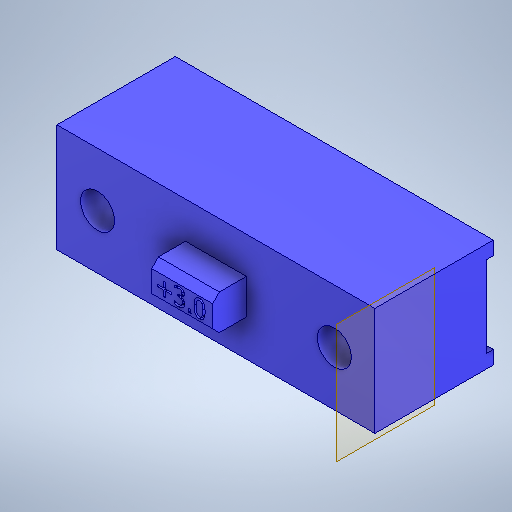
# Autodesk Inventor part: Bearing Spacer_V2_3mm
Saved by Autodesk Inventor 2025.4 (Build 294407000, 407)
## iProperties
Created: 2026-06-01
Part Number: Bearing Spacer_V2_3mm
Material: 일반
Document SubType Name: Modeling
Designer: dalbi
Density: 1 g/cm^3
Appearance: 기본값
Author: dalbi
Autodesk Inventor part; units mm, degrees
ref_plane "YZ Plane" through (0, 0, 0) normal (1, 0, 0) x (0, 1, 0)
ref_plane "XZ Plane" through (0, 0, 0) normal (0, 1, 0) x (-1, 0, 0)
ref_plane "XY Plane" through (0, 0, 0) normal (0, 0, 1) x (1, 0, 0)
ref_plane "작업 평면1" through (23.5, -8, -2) normal (1, 0, 0) x (0, 0, -1)
sketch "스케치1" plane through (23.5, -8, -2) normal (1, 0, 0) x (0, 0, -1)
  line L0 (0, 16) -> (-8.15, 16) projected
  line L1 (-8.15, 16) -> (-8.15, 10.6) projected
  line L2 (-8.15, 10.6) -> (-12.15, 10.6) projected
  line L3 (-13.15, 9.6) -> (-12.15, 10.6) projected
  line L4 (-13.15, 9.6) -> (-13.15, 6.4) projected
  line L5 (-12.15, 5.4) -> (-13.15, 6.4) projected
  line L6 (-12.15, 5.4) -> (-8.15, 5.4) projected
  line L7 (-8.15, 5.4) -> (-8.15, 0) projected
  line L8 (-8.15, 0) -> (0, 0) projected
  line L9 (0, 16) -> (9.35, 16)
  line L10 (9.35, 16) -> (9.35, 15)
  line L11 (0, 0) -> (9.35, 0)
  line L12 (9.35, 0) -> (9.35, 1)
  line L13 (0, 16) -> (-8.15, 16)
  line L14 (-8.15, 10.6) -> (-12.15, 10.6) projected
  line L15 (-8.15, 10.6) -> (-12.15, 10.6)
  line L16 (-12.15, 10.6) -> (-13.15, 9.6)
  line L17 (-13.15, 6.4) -> (-12.15, 5.4)
  line L18 (8.35, 14) -> (9.35, 14)
  line L19 (9.35, 14) -> (9.35, 15)
  line L20 (8.35, 2) -> (9.35, 2)
  line L21 (9.35, 2) -> (9.35, 1)
  line L22 (8.35, 14) -> (8.35, 2)
  point P0 (-2, 8)
  point P1 (4.35, 10.6)
  point P2 (4.35, 5.4)
  dimension "d1" = 9.35
  dimension "d13" = 9.35
  constraints: 26 end point, 5 perpendicular, 4 horizontal, 2 collinear, 2 point on line
  measures "d1" distance of L0.start L9.end
  measures "d13" distance of L8.end L11.end
sketch "스케치2" plane through (-23.5, 8, 6.15) normal (0, 0, 1) x (1, 0, 0)
  arc A0 (7.9209, -9.6) -> (7.9209, -6.4) centre (6, -8) ccw projected
  line L0 (39.0791, -9.6) -> (7.9209, -9.6) projected
  circle A1 centre (6, -8) radius 2.5
  circle A2 centre (41, -8) radius 2.5 projected
  circle A3 centre (41, -8) radius 2.5
  point P0 (23.5, -8)
  point P1 (7.9209, -6.4)
  constraints: 2 coincident, 1 centre point, 4 other
extrude "돌출1" add sketch "스케치1" against normal up to surface (47 mm away)
extrude "돌출2" cut sketch "스케치2" along normal mid plane 50
sketch "스케치3" plane through (-15.5791, 1.6, 11.15) normal (0, 0, 1) x (1, 0, 0)
  line L0 (15.5791, -14.4593) -> (15.5791, 15.5737)
  line L1 (-7.9209, 4.4) -> (-7.9209, -7.6) projected
  line L2 (-7.9209, 4.4) -> (11.0791, 4.4)
  line L3 (11.0791, 4.4) -> (11.0791, -7.6)
  line L4 (11.0791, -7.6) -> (-7.9209, -7.6)
  line L5 (-7.9209, -7.6) -> (-7.9209, 4.4)
  line L6 (39.0791, 4.4) -> (39.0791, -7.6)
  line L7 (39.0791, 4.4) -> (20.0791, 4.4)
  line L8 (20.0791, 4.4) -> (20.0791, -7.6)
  line L9 (20.0791, -7.6) -> (39.0791, -7.6)
  line L10 (39.0791, -7.6) -> (39.0791, 4.4)
  point P0 (15.5791, -1.6)
  dimension "d9" = 19
  constraints: 20 end point, 5 symmetric about line, 2 parallel, 1 horizontal, 1 perpendicular, 1 vertical
  measures "d9" distance of L1.start L2.end
extrude "돌출3" cut sketch "스케치3" against normal up to surface (5 mm away)
sketch "스케치4" plane through (-4.5, 1.6, 11.15) normal (0, 0, 1) x (1, 0, 0)
  line L0 (0.6181, -0.2528) -> (7.2489, -0.2528) construction
  line L1 (7.2489, -0.2528) -> (7.2489, -2.6222) construction
  line L2 (7.2489, -2.6222) -> (0.6181, -2.6222) construction
  line L3 (0.6181, -2.6222) -> (0.6181, -0.2528) construction
  line L4 (2.8925, -1.8707) -> (2.0321, -1.8707)
  line L5 (2.0321, -1.8707) -> (2.0321, -2.7311)
  line L6 (2.0321, -2.7311) -> (1.7481, -2.7311)
  line L7 (1.7481, -2.7311) -> (1.7481, -1.8707)
  line L8 (1.7481, -1.8707) -> (0.8877, -1.8707)
  line L9 (0.8877, -1.8707) -> (0.8877, -1.5969)
  line L10 (0.8877, -1.5969) -> (1.7481, -1.5969)
  line L11 (1.7481, -1.5969) -> (1.7481, -0.7365)
  line L12 (1.7481, -0.7365) -> (2.0321, -0.7365)
  line L13 (2.0321, -0.7365) -> (2.0321, -1.5969)
  line L14 (2.0321, -1.5969) -> (2.8925, -1.5969)
  line L15 (2.8925, -1.5969) -> (2.8925, -1.8707)
  spline S0 degree 2 poles (4.0308, -0.5472) (3.9382, -0.5472) (3.755, -0.5925) (3.6665, -0.6274) knots 0 0 0 1 2 2 2
  spline S1 degree 2 poles (3.6665, -0.6274) (3.5841, -0.6624) (3.4627, -0.7365) (3.4154, -0.7695) knots 0 0 0 1 2 2 2
  line L16 (3.4154, -0.7695) -> (3.3948, -0.7695)
  line L17 (3.3948, -0.7695) -> (3.3948, -0.4093)
  spline S2 degree 2 poles (3.3948, -0.4093) (3.5059, -0.3496) (3.8867, -0.2528) (4.0576, -0.2528) knots 0 0 0 1 2 2 2
  spline S3 degree 2 poles (4.0576, -0.2528) (4.2305, -0.2528) (4.4878, -0.3228) (4.5927, -0.3969) knots 0 0 0 1 2 2 2
  spline S4 degree 2 poles (4.5927, -0.3969) (4.7039, -0.4772) (4.8191, -0.7098) (4.8191, -0.8662) knots 0 0 0 1 2 2 2
  spline S5 degree 2 poles (4.8191, -0.8662) (4.8191, -1.0762) (4.5433, -1.3932) (4.3498, -1.4343) knots 0 0 0 1 2 2 2
  line L18 (4.3498, -1.4343) -> (4.3498, -1.459)
  spline S6 degree 2 poles (4.3498, -1.459) (4.4301, -1.4755) (4.6133, -1.5496) (4.6915, -1.6237) knots 0 0 0 1 2 2 2
  spline S7 degree 2 poles (4.6915, -1.6237) (4.7697, -1.6957) (4.8685, -1.9263) (4.8685, -2.093) knots 0 0 0 1 2 2 2
  spline S8 degree 2 poles (4.8685, -2.093) (4.8685, -2.2638) (4.7512, -2.5541) (4.6442, -2.6652) knots 0 0 0 1 2 2 2
  spline S9 degree 2 poles (4.6442, -2.6652) (4.533, -2.7805) (4.2181, -2.8999) (4.0184, -2.8999) knots 0 0 0 1 2 2 2
  spline S10 degree 2 poles (4.0184, -2.8999) (3.827, -2.8999) (3.4524, -2.8072) (3.3248, -2.7434) knots 0 0 0 1 2 2 2
  line L19 (3.3248, -2.7434) -> (3.3248, -2.3832)
  line L20 (3.3248, -2.3832) -> (3.3495, -2.3832)
  spline S11 degree 2 poles (3.3495, -2.3832) (3.4565, -2.4614) (3.8188, -2.6055) (3.9979, -2.6055) knots 0 0 0 1 2 2 2
  spline S12 degree 2 poles (3.9979, -2.6055) (4.1028, -2.6055) (4.3128, -2.5396) (4.3828, -2.4635) knots 0 0 0 1 2 2 2
  spline S13 degree 2 poles (4.3828, -2.4635) (4.4507, -2.3873) (4.5227, -2.2062) (4.5227, -2.0683) knots 0 0 0 1 2 2 2
  spline S14 degree 2 poles (4.5227, -2.0683) (4.5227, -1.9304) (4.4425, -1.7513) (4.3704, -1.6998) knots 0 0 0 1 2 2 2
  spline S15 degree 2 poles (4.3704, -1.6998) (4.2984, -1.6484) (4.1028, -1.6093) (3.9876, -1.6093) knots 0 0 0 1 2 2 2
  line L21 (3.9876, -1.6093) -> (3.8435, -1.6093)
  line L22 (3.8435, -1.6093) -> (3.8435, -1.3273)
  line L23 (3.8435, -1.3273) -> (3.9567, -1.3273)
  spline S16 degree 2 poles (3.9567, -1.3273) (4.1852, -1.3273) (4.4733, -1.1091) (4.4733, -0.9012) knots 0 0 0 1 2 2 2
  spline S17 degree 2 poles (4.4733, -0.9012) (4.4733, -0.8045) (4.3992, -0.6666) (4.3396, -0.6254) knots 0 0 0 1 2 2 2
  spline S18 degree 2 poles (4.3396, -0.6254) (4.2757, -0.5822) (4.1193, -0.5472) (4.0308, -0.5472) knots 0 0 0 1 2 2 2
  line L24 (5.7969, -2.8463) -> (5.3893, -2.8463)
  line L25 (5.3893, -2.8463) -> (5.3893, -2.3606)
  line L26 (5.3893, -2.3606) -> (5.7969, -2.3606)
  line L27 (5.7969, -2.3606) -> (5.7969, -2.8463)
  spline S19 degree 2 poles (7.8902, -1.5763) (7.8902, -2.2597) (7.4929, -2.8999) (7.0792, -2.8999) knots 0 0 0 1 2 2 2
  spline S20 degree 2 poles (7.0792, -2.8999) (6.6593, -2.8999) (6.2662, -2.2474) (6.2662, -1.5784) knots 0 0 0 1 2 2 2
  spline S21 degree 2 poles (6.2662, -1.5784) (6.2662, -0.8909) (6.6634, -0.2549) (7.0792, -0.2549) knots 0 0 0 1 2 2 2
  spline S22 degree 2 poles (7.0792, -0.2549) (7.4971, -0.2549) (7.8902, -0.9136) (7.8902, -1.5763) knots 0 0 0 1 2 2 2
  spline S23 degree 2 poles (7.4538, -2.3503) (7.5032, -2.2247) (7.5444, -1.8378) (7.5444, -1.5763) knots 0 0 0 1 2 2 2
  spline S24 degree 2 poles (7.5444, -1.5763) (7.5444, -1.3149) (7.5032, -0.93) (7.4518, -0.8003) knots 0 0 0 1 2 2 2
  spline S25 degree 2 poles (7.4518, -0.8003) (7.4003, -0.6707) (7.2212, -0.5369) (7.0792, -0.5369) knots 0 0 0 1 2 2 2
  spline S26 degree 2 poles (7.0792, -0.5369) (6.9372, -0.5369) (6.754, -0.6707) (6.7005, -0.8045) knots 0 0 0 1 2 2 2
  spline S27 degree 2 poles (6.7005, -0.8045) (6.649, -0.9341) (6.612, -1.3293) (6.612, -1.5784) knots 0 0 0 1 2 2 2
  spline S28 degree 2 poles (6.612, -1.5784) (6.612, -1.846) (6.6449, -2.2041) (6.6984, -2.3441) knots 0 0 0 1 2 2 2
  spline S29 degree 2 poles (6.6984, -2.3441) (6.7478, -2.4758) (6.931, -2.6179) (7.0792, -2.6179) knots 0 0 0 1 2 2 2
  spline S30 degree 2 poles (7.0792, -2.6179) (7.2192, -2.6179) (7.4024, -2.4841) (7.4538, -2.3503) knots 0 0 0 1 2 2 2
  point P0 (4.5, -1.6)
  constraints: 2 other
extrude "돌출4" cut sketch "스케치4" against normal blind 5
